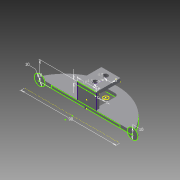
# Autodesk Inventor part: ZFoot
Saved by Autodesk Inventor 2014 SP1 (Build 180222100, 222)
## iProperties
Created: 2014-07-13
Part Number: ZFoot
Material: Generic
Document SubType Name: Modeling
Designer: Erin
Density: 1 g/cm^3
Appearance: Default
Author: Erin
Autodesk Inventor part; units mm, degrees
ref_plane "YZ Plane" through (0, 0, 0) normal (1, 0, 0) x (0, 1, 0)
ref_plane "XZ Plane" through (0, 0, 0) normal (0, 1, 0) x (-1, 0, 0)
ref_plane "XY Plane" through (0, 0, 0) normal (0, 0, 1) x (1, 0, 0)
sketch "Sketch1" plane through (0, 0, 0) normal (0, 1, 0) x (-1, 0, 0)
  line L0 (-9, 10.6795) -> (9, 10.6795)
  line L1 (9, 10.6795) -> (9, -4.7118)
  line L2 (9, -4.7118) -> (-9, -4.7118)
  line L3 (-9, -4.7118) -> (-9, 10.6795)
  line L4 (-9, 7.6795) -> (9, 7.6795)
  line L5 (-31.4348, -4.7118) -> (33.5217, -4.7118)
  line L6 (33.5217, -4.7118) -> (33.5217, -7.3205)
  line L7 (33.5217, -7.3205) -> (-31.4348, -7.3205)
  line L8 (-31.4348, -7.3205) -> (-31.4348, -4.7118)
  circle A0 centre (-43.3004, -6.0161) radius 5
  circle A1 centre (44.4458, -6.0161) radius 5
  point P0 (0, 0)
  point P1 (0, 7.6795)
  dimension "d6" = 3
  dimension "d7" = 18
  dimension "d8" = 18
  dimension "d34" = 10
  dimension "d35" = 10
  constraints: 18 end point, 4 parallel, 3 perpendicular, 2 centre point, 2 horizontal, 2 point on line, 1 collinear, 1 midpoint, 1 vertical alignment
  measures "d6" distance between parallel lines of L4 L0
  measures "d7" distance between parallel lines of L7 L0
  measures "d8" distance of L0.start L0.end
  measures "d34" diameter of A0
  measures "d35" diameter of A1
extrude "Extrusion2" add sketch "Sketch1" along normal blind 3 contours L0 L1 L4 L3 | L4 L1 L2 L3 | L2 L5 L6 L7 L8
extrude "Extrusion3" add sketch "Sketch1" along normal blind 23 contours L0 L1 L4 L3
sketch "Sketch2" plane through (9, 3, 7.6795) normal (0, 0, -1) x (-1, 0, 0)
  line L0 (18, 0) -> (0, 0) projected
  line L1 (0, 20) -> (18, 20) projected
  circle A0 centre (9, 15) radius 2.25
  circle A1 centre (9, 5) radius 2.25
  circle A2 centre (9, 5) radius 4.25
  circle A3 centre (9, 15) radius 4.25
  point P0 (9, -3)
  point P1 (9, 20)
  point P2 (9, 0)
  dimension "d15" = 4.5
  dimension "d16" = 4.5
  dimension "d17" = 5
  dimension "d18" = 5
  dimension "d19" = 2
  dimension "d20" = 2
  constraints: 4 centre point, 2 midpoint, 2 vertical alignment
  measures "d15" diameter of A0
  measures "d16" diameter of A1
  measures "d17" distance from line of A1.centre L0
  measures "d18" distance from line of A0.centre L1
  measures "d19" radial gap between concentric circles of A3 A0
  measures "d20" radial gap between concentric circles of A1 A2
extrude "Extrusion4" cut sketch "Sketch2" against normal blind 3 contours A0 | A1
extrude "Extrusion5" add sketch "Sketch2" along normal blind 3
sketch "Sketch3" plane through (31.4348, 0, -7.3205) normal (0, 0, -1) x (-1, 0, 0)
  line L0 (64.9565, 0) -> (0, 0) projected
  line L1 (0, 3) -> (64.9565, 3) projected
  line L2 (24.4348, 23.1251) -> (38.4348, 23.1251)
  line L3 (38.4348, 23.1251) -> (38.4348, 3)
  line L4 (38.4348, 3) -> (24.4348, 3)
  line L5 (24.4348, 3) -> (24.4348, 23.1251)
  circle A0 centre (31.4348, 18) radius 2.25 projected
  circle A1 centre (31.4348, 8) radius 2.25 projected
  line L6 (0, 0) -> (0, 3) projected
  line L7 (-12.5217, -12.4797) -> (77.4783, -12.4797) construction
  arc A2 (77.4783, 0) -> (-12.5217, 0) centre (32.4783, -18.9639) ccw
  line L8 (-12.5217, 0) -> (77.4783, 0)
  point P0 (31.4348, 0)
  point P1 (32.4783, -12.4797)
  point P2 (32.4783, 0)
  dimension "d27" = 7
  dimension "d28" = 7
  dimension "d29" = 90
  constraints: 12 end point, 3 parallel, 2 midpoint, 2 perpendicular, 2 point on circle, 1 centre point, 1 horizontal, 1 point on line, 1 vertical alignment
  measures "d27" distance from line of A0.centre L5
  measures "d28" distance from line of A0.centre L3
  measures "d29" distance of L7.start L7.end
extrude "Extrusion6" add sketch "Sketch3" against normal blind 3 contours L0 L8 A2
fillet "Fillet1" radius 3 2 edges at (-46.0435, 0, -5.8205) (43.9565, 0, -5.8205)
fillet "Fillet2" radius 3 4 edges at (7, 3, -5.8205) (-7, 3, -5.8205) (-7, 23.1251, -5.8205) (7, 23.1251, -5.8205)
extrude "Extrusion8" add sketch "Sketch1" along normal blind 0.6 contours A0 | A1
body "Solid2"
